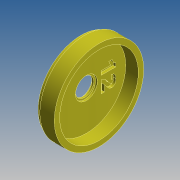
# Autodesk Inventor part: P114PorteLentille20mm
Saved by Autodesk Inventor 2015 SP1 (Build 190203100, 203)
## iProperties
Created: 2016-11-02
Part Number: P114PorteLentille20mm
Material: ABS Plastic
Document SubType Name: Modeling
Designer: serge.amoos
Density: 1.06 g/cm^3
Appearance: Canary
Author: serge.amoos
Autodesk Inventor part; units mm, degrees
ref_plane "YZ Plane" through (0, 0, 0) normal (1, 0, 0) x (0, 1, 0)
ref_plane "XZ Plane" through (0, 0, 0) normal (0, 1, 0) x (-1, 0, 0)
ref_plane "XY Plane" through (0, 0, 0) normal (0, 0, 1) x (1, 0, 0)
sketch "Sketch1" plane through (0, 0, 0) normal (0, 0, 1) x (1, 0, 0)
  line L0 (-12, 0) -> (2, 0) construction
  line L1 (0, -4.98) -> (0, 29.88) construction
  line L2 (-9, 5.1) -> (-9, 6.1)
  line L3 (-9, 6.1) -> (-10, 6.1)
  line L4 (-10, 6.1) -> (-10, 23.9)
  line L5 (-10, 23.9) -> (-8, 23.9)
  line L6 (-8, 23.9) -> (-8, 24.9)
  line L7 (-8, 24.9) -> (0, 24.9)
  line L8 (0, 21.9) -> (-7, 21.9)
  line L9 (-7, 21.9) -> (-7, 6.1)
  line L10 (0, 24.9) -> (0, 21.9)
  line L11 (-9, 5.1) -> (-8, 5.1)
  line L12 (-8, 5.1) -> (-8, 6.1)
  line L13 (-8, 6.1) -> (-7, 6.1)
  point P0 (0, 0)
  dimension "d0" = 49.8
  dimension "d1" = 47.8
  dimension "d3" = 1
  dimension "d4" = 2
  dimension "d7" = 3
  dimension "d8" = 3
  dimension "d10" = 10
  dimension "d17" = 12.2
  dimension "d20" = 1
  dimension "d21" = 1
  constraints: 24 end point, 8 perpendicular, 2 collinear, 1 horizontal, 1 point on line, 1 vertical
  measures "d0" diameter of L7 L0
  measures "d1" diameter of L5 L0
  measures "d3" distance between parallel lines of L2 L4
  measures "d4" distance between parallel lines of L4 L6
  measures "d7" distance between parallel lines of L8 L7
  measures "d8" distance between parallel lines of L9 L4
  measures "d10" distance between parallel lines of L1 L4
  measures "d17" diameter of L3 L0
  measures "d20" distance between parallel lines of L2 L12
  measures "d21" distance between parallel lines of L11 L13
revolve "Revolution1" add sketch "Sketch1" angle 360 about axis through (-10, 0, 0) along (1, 0, 0)
sketch "Sketch2" plane through (-7, 0, 0) normal (1, 0, 0) x (0, 0, -1)
  line L0 (0, -34.86) -> (0, 34.86) construction
  line L1 (34.86, 0) -> (-34.86, 0) construction
  line L2 (-6.2231, 15.472) -> (6.2231, 15.472) construction
  line L3 (6.2231, 15.472) -> (6.2231, 9.2435) construction
  line L4 (6.2231, 9.2435) -> (-6.2231, 9.2435) construction
  line L5 (-6.2231, 9.2435) -> (-6.2231, 15.472) construction
  line L6 (-1.9634, 16.4271) -> (-1.9634, 8.2885)
  line L7 (-1.9634, 8.2885) -> (-4.2117, 8.2885)
  line L8 (-4.2117, 8.2885) -> (-4.2117, 13.6244)
  spline S0 degree 2 poles (-4.2117, 13.6244) (-4.7584, 13.2086) (-5.7748, 12.7004) (-6.5448, 12.4617) knots 0 0 0 1 2 2 2
  line L9 (-6.5448, 12.4617) -> (-6.5448, 14.2865)
  spline S1 degree 2 poles (-6.5448, 14.2865) (-5.4129, 14.6484) (-4.1578, 15.6725) (-3.8037, 16.4271) knots 0 0 0 1 2 2 2
  line L10 (-3.8037, 16.4271) -> (-1.9634, 16.4271)
  line L11 (6.9605, 8.2885) -> (0.2926, 8.2885)
  spline S2 degree 2 poles (0.2926, 8.2885) (0.4081, 9.274) (1.5707, 11.0142) (3.1723, 12.1999) knots 0 0 0 1 2 2 2
  spline S3 degree 2 poles (3.1723, 12.1999) (4.1424, 12.9237) (4.6891, 13.6783) (4.6891, 14.017) knots 0 0 0 1 2 2 2
  spline S4 degree 2 poles (4.6891, 14.017) (4.6891, 14.3866) (4.1501, 14.9025) (3.7421, 14.9025) knots 0 0 0 1 2 2 2
  spline S5 degree 2 poles (3.7421, 14.9025) (3.3109, 14.9025) (2.7719, 14.3712) (2.6795, 13.6937) knots 0 0 0 1 2 2 2
  line L12 (2.6795, 13.6937) -> (0.4543, 13.8708)
  spline S6 degree 2 poles (0.4543, 13.8708) (0.5852, 14.8101) (1.2859, 15.865) (2.5563, 16.4271) (3.6805, 16.4271) knots 0 0 0 1 2 3 3 3
  spline S7 degree 2 poles (3.6805, 16.4271) (4.8508, 16.4271) (6.1598, 15.8881) (6.9066, 14.787) (6.9066, 14.094) knots 0 0 0 1 2 3 3 3
  spline S8 degree 2 poles (6.9066, 14.094) (6.9066, 13.3626) (6.052, 12.0305) (4.9201, 11.2297) knots 0 0 0 1 2 2 2
  spline S9 degree 2 poles (4.9201, 11.2297) (4.2502, 10.7678) (3.796, 10.3982) (3.488, 10.0979) knots 0 0 0 1 2 2 2
  line L13 (3.488, 10.0979) -> (6.9605, 10.0979)
  line L14 (6.9605, 10.0979) -> (6.9605, 8.2885)
  point P0 (0, 0)
  point P1 (0, 15.472)
  constraints: 1 midpoint, 1 point on line, 2 other
extrude "Extrusion1" cut sketch "Sketch2" against normal blind 1.5
body "Solid1"
